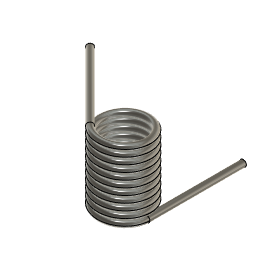
Joint stacked torsion module (Autodesk Fusion 360 archive; units mm, degrees)
design "Torsion spring right wind  0.8mm* wire 6mm OD 8mm length"
Autodesk Fusion 360 part; units mm, degrees
note: some values were not read from the file. Chosen so that the rebuilt part matches the saved one: the hand of a thread or coil; which face or edge a step refers to.
coil "CoilPrimitive1" add diameter 5.8 section circle size 0.7 inside turns 10.375 pitch 0.72289 left hand placed x (1, 0, 0) y (0, 1, 0) z (0, 0, 1) at (0, 0, 0) makes body 1
extrude "Extrude1" add 1 faces at (-1.7088, -1.7088, 7.3962) along direction (-0.707107, 0.707107, 0) blind 10.5 on bodies 1 bodies 1
extrude "Extrude2" add 1 faces at (2.6814, 0, 0.1001) along direction (0, 1, 0) blind 10.5 separate body on bodies 1 makes body 2
copy_body "Body->Comp1" bodies 1 removing the originals makes body 3 in component "Main-spring"
copy_body "Body->Comp2" bodies 2 removing the originals makes body 4 in component "Actuated-leg"
component "Main-spring" placed x (1, 0, 0) y (0, 1, 0) z (0, 0, 1) at (0, 0, 0)
component "Actuated-leg" placed x (1, 0, 0) y (0, 1, 0) z (0, 0, 1) at (0, 0, 0)
equation "d1 = outer_diameter"
equation "d2 = wire_diameter"
equation "d4 = turns - ( extension * 0.5 / 180 deg )"
equation "d5 = height - 0.5 mm"
equation "d6 = prong_length"
equation "d8 = prong_length"
equation "wire_diameter = 0.7 mm"
equation "height = 8 mm"
equation "outer_diameter = 5.8 mm"
equation "extension = 45 deg"
equation "turns = 10.5" comment "Extra half a turn to make it U shaped."
equation "prong_length = 10.5 mm"
